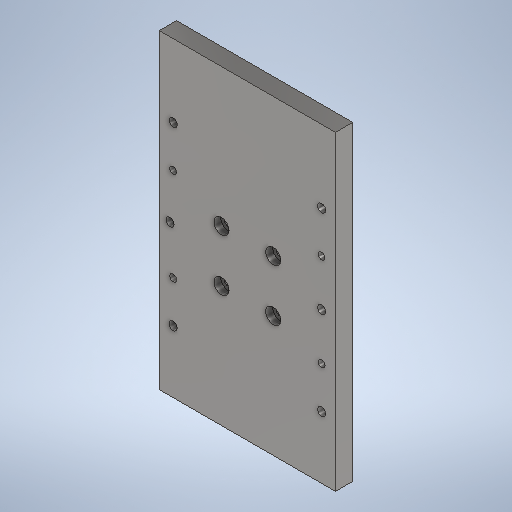
# Autodesk Inventor part: Ball_Spacer
Saved by Autodesk Inventor 2025.2 (Build 292293000, 293)
## iProperties
Created: 2024-12-11
Part Number: Ball_Spacer
Material: Steel, Carbon
Document SubType Name: Modeling
Designer: konch
Density: 7.85 g/cm^3
Appearance: Semi-Polished
Mass: 44.37 g
Surface Area: 116.34 cm^2
Volume: 44.37 cm^3
Author: konch
Autodesk Inventor part; units mm, degrees
ref_plane "YZ Plane" through (0, 0, 0) normal (1, 0, 0) x (0, 1, 0)
ref_plane "XZ Plane" through (0, 0, 0) normal (0, 1, 0) x (-1, 0, 0)
ref_plane "XY Plane" through (0, 0, 0) normal (0, 0, 1) x (1, 0, 0)
sketch "Sketch1" plane through (0, 0, 0) normal (0, 0, 1) x (1, 0, 0)
  line L0 (0, 0) -> (51, 0)
  line L1 (51, 0) -> (51, 90)
  line L2 (51, 90) -> (0, 90)
  line L3 (0, 90) -> (0, 0)
  dimension "d0" = 51
  dimension "d1" = 90
  constraints: 8 end point, 3 perpendicular, 1 horizontal
  measures "d0" distance of L0.start L0.end
  measures "d1" distance of L0.end L1.end
extrude "Extrusion1" add sketch "Sketch1" along normal blind 5
sketch "Sketch2" plane through (0, 0, 5) normal (0, 0, 1) x (1, 0, 0)
  line L0 (0, 0) -> (51, 0) construction
  line L1 (25.5, 0) -> (25.5, 90) construction
  line L2 (51, 90) -> (0, 90) construction
  line L3 (51, 0) -> (51, 90) construction
  line L4 (51, 45) -> (0, 45) construction
  line L5 (25.5, 45) -> (25.5, 35) construction
  line L6 (25.5, 35) -> (18, 35) construction
  line L7 (18, 35) -> (18, 50) construction
  line L8 (18, 50) -> (33, 50) construction
  line L9 (33, 50) -> (33, 35) construction
  dimension "d23" = 10
  dimension "d24" = 7.5
  dimension "d25" = 15
  dimension "d26" = 15
  constraints: 14 end point, 5 coincident, 4 midpoint, 4 perpendicular, 2 point on line, 1 horizontal
  measures "d23" distance of L5.start L5.end
  measures "d24" distance of L5.end L6.end
  measures "d25" distance of L6.end L7.end
  measures "d26" distance of L7.end L8.end
sketch "Sketch3" plane through (0, 0, 0) normal (0, 0, -1) x (-1, 0, 0)
  line L0 (-51, 90) -> (0, 90) projected
  line L1 (-51, 90) -> (-41, 90)
  line L2 (-41, 90) -> (-41, 0)
  line L3 (0, 90) -> (-10.0159, 90)
  line L4 (-10.0159, 90) -> (-10.0159, 0)
  line L5 (0, 0) -> (-51, 0) projected
  line L6 (-51, 90) -> (-51, 79)
  line L7 (-51, 79) -> (0, 79)
  line L8 (-51, 0) -> (-51, 8)
  line L9 (-51, 0) -> (-51, 90) projected
  line L10 (-51, 8) -> (0, 8)
  line L11 (-51, 90) -> (-46, 90)
  line L12 (-51, 79) -> (-46, 79)
  line L13 (-46, 90) -> (-46, 69)
  line L14 (-10.0159, 45) -> (-4.0159, 45)
  line L15 (0, 90) -> (0, 0) projected
  line L16 (-41, 90) -> (-41, 48.5) construction
  line L17 (-47, 45) -> (-4.0159, 45)
  line L18 (-47, 43.5703) -> (-3.108, 43.5703)
  line L19 (-41, 90) -> (-47, 90)
  line L20 (-47, 90) -> (-47, 0)
  line L21 (-47, 0) -> (-47, 18)
  line L22 (-10.0159, 0) -> (-4.0159, 0)
  line L23 (-4.0159, 0) -> (-4.0159, 18)
  line L24 (-10.0159, 90) -> (-4.0159, 90)
  line L25 (-4.0159, 90) -> (-4.0159, 69)
  point P0 (-5, 69)
  point P1 (-46, 18)
  point P2 (-5, 18)
  point P3 (-48.5, 90)
  point P4 (-25.054, 43.5703)
  point P5 (-25.508, 45)
  point P6 (-47, 69)
  dimension "d8" = 11
  dimension "d9" = 8
  dimension "d15" = 21
  dimension "d38" = 5
  dimension "d41" = 6
  dimension "d47" = 10
  dimension "d48" = 10.016
  dimension "d50" = 1.5
  dimension "d54" = 6
  dimension "d55" = 18
  dimension "d56" = 6
  dimension "d57" = 6
  constraints: 44 end point, 14 point on line, 7 coincident, 6 midpoint, 6 perpendicular, 2 horizontal, 2 vertical, 1 collinear, 1 parallel
  measures "d8" distance of L0.start L6.end
  measures "d9" distance of L5.end L8.end
  measures "d15" distance of L11.end L13.end
  measures "d38" distance from line of L2 point (-46, 18)
  measures "d41" distance of L14.end L14.start
  measures "d47" distance of L1.end L0.start
  measures "d50" distance of point (-25.054, 43.57) point (-25.508, 45)
  measures "d54" distance of L1.end L19.end
  measures "d55" distance of L20.end L21.end
  measures "d56" distance of L4.end L22.end
  measures "d57" distance of L3.end L24.end
hole "Hole1" at (47, 69, 0) at (47, 43.5703, 0) at (47, 18, 0) at (4.0159, 18, 0) at (3.108, 43.5703, 0) at (4.0159, 69, 0) direction (0, 0, 1) diameter 2.4 end through all counterbore diameter 4.4 counterbore depth 2
hole "Hole2" at (33, 50, 5) at (18, 50, 5) at (18, 35, 5) at (33, 35, 5) direction (0, 0, -1) diameter 2.4 end through all counterbore diameter 4.4 counterbore depth 2
chamfer "Chamfer1" distance 0.3 angle 45 4 edges at (33, 51.2, 0) (33, 36.2, 0) (18, 51.2, 0) (18, 36.2, 0)
sketch "Sketch4" plane through (0, 0, 0) normal (0, 0, -1) x (-1, 0, 0)
  circle A0 centre (-47, 69) radius 1.2 projected
  line L0 (-47, 69) -> (-47, 57)
  circle A1 centre (-47, 18) radius 1.2 projected
  line L1 (-47, 18) -> (-47, 30)
  circle A2 centre (-4.0159, 18) radius 1.2 projected
  line L2 (-4.0159, 18) -> (-4.0159, 30)
  circle A3 centre (-4.0159, 69) radius 1.2 projected
  line L3 (-4.0159, 69) -> (-4.0159, 57)
  point P0 (0, 0)
  dimension "d58" = 12
  dimension "d59" = 12
  dimension "d60" = 12
  dimension "d61" = 12
  constraints: 8 end point, 4 coincident, 4 vertical
  measures "d58" distance of L0.start L0.end
  measures "d59" distance of L1.start L1.end
  measures "d60" distance of L2.start L2.end
  measures "d61" distance of L3.start L3.end
hole "Hole3" at (47, 57, 0) at (4.0159, 57, 0) at (4.0159, 30, 0) at (47, 30, 0) direction (0, 0, 1) diameter 2 end through all
chamfer "Chamfer2" distance 0.3 angle 45 4 edges at (47, 56, 0) (47, 29, 0) (4.0159, 29, 0) (4.0159, 56, 0)
body "Solid1"
